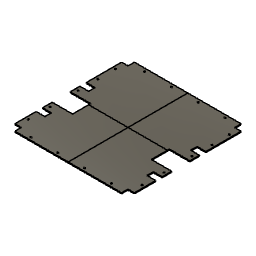
Legacy bottom panel v3 (Autodesk Fusion 360 design; units mm, degrees)
Autodesk Fusion 360 part; units mm, degrees
sketch "Sketch1" plane through (0, 0, 0) normal (0, 0, 1) x (1, 0, 0)
  line L0 (0, 0) -> (410, 0)
  line L1 (410, 0) -> (410, -410)
  line L2 (410, -410) -> (0, -410)
  line L3 (0, -410) -> (0, 0)
  dimension "d1" = 410
  dimension "d2" = 410
  constraint horizontal L0
  constraint vertical L1
  constraint horizontal L2
  constraint vertical L3
  constraint coincident L0.start L3.end
  measures "d1" distance of L0.start L0.end
  measures "d2" distance of L0.start L2.end
extrude "Extrude1" add sketch "Sketch1" along normal blind 3 makes body 1
move_body "Move1" bodies 1 to x (1, 0, 0) y (0, 1, 0) z (0, 0, 1) at (0, 205, 0)
sketch "Sketch2" plane through (0, 0, 3) normal (0, 0, 1) x (-1, 0, 0)
  line L0 (0, 205) -> (-410, 205)
  line L1 (-410, 205) -> (-410, -205)
  line L2 (-410, -205) -> (0, -205)
  line L3 (0, -205) -> (0, 205)
  line L4 (0, -205) -> (-22, -205)
  line L5 (-22, -205) -> (-22, -183)
  line L6 (-22, -183) -> (0, -183)
  line L7 (0, -183) -> (0, -205)
  line L8 (-410, -205) -> (-388, -205)
  line L9 (-388, -205) -> (-388, -183)
  line L10 (-388, -183) -> (-410, -183)
  line L11 (-410, -183) -> (-410, -205)
  line L12 (0, 205) -> (-22, 205)
  line L13 (-22, 205) -> (-22, 183)
  line L14 (-22, 183) -> (0, 183)
  line L15 (0, 183) -> (0, 205)
  line L16 (-410, 205) -> (-388, 205)
  line L17 (-388, 205) -> (-388, 183)
  line L18 (-388, 183) -> (-410, 183)
  line L19 (-410, 183) -> (-410, 205)
  dimension "d5" = 22
  dimension "d6" = 22
  dimension "d9" = 22
  dimension "d10" = 22
  dimension "d11" = 22
  dimension "d12" = 22
  dimension "d13" = 22
  dimension "d14" = 22
  constraint horizontal L4
  constraint vertical L5
  constraint horizontal L6
  constraint vertical L7
  constraint coincident L2.end L3.start
  constraint horizontal L8
  constraint vertical L9
  constraint horizontal L10
  constraint vertical L11
  constraint coincident L1.end L2.start
  constraint horizontal L12
  constraint vertical L13
  constraint horizontal L14
  constraint vertical L15
  constraint coincident L0.start L3.end
  constraint horizontal L16
  constraint vertical L17
  constraint horizontal L18
  constraint vertical L19
  constraint coincident L0.end L1.start
  measures "d5" distance of L2.end L4.end
  measures "d6" distance of L2.end L6.end
  measures "d9" distance of L1.end L8.end
  measures "d10" distance of L1.end L10.end
  measures "d11" distance of L0.start L12.end
  measures "d12" distance of L0.start L14.end
  measures "d13" distance of L0.end L16.end
  measures "d14" distance of L0.end L18.end
extrude "Extrude2" cut sketch "Sketch2" against normal blind 10 contours L2 L3 L4 L5 L6 L7 bodies 1
extrude "Extrude3" cut sketch "Sketch2" against normal blind 10 contours L0 L3 L12 L13 L14 L15 | L2 L3 L4 L5 L6 L7 | L1 L2 L8 L9 L10 L11 bodies 1
extrude "Extrude4" cut sketch "Sketch2" against normal blind 10 contours L0 L1 L16 L17 L18 L19 bodies 1
sketch "Sketch6" plane through (0, 0, 3) normal (0, 0, 1) x (-1, 0, 0)
  line L0 (-388, 205) -> (-388, 183)
  line L1 (-388, 183) -> (-410, 183)
  line L2 (-410, 183) -> (-410, -183)
  line L3 (-410, -183) -> (-388, -183)
  line L4 (-388, -183) -> (-388, -205)
  line L5 (-388, -205) -> (-22, -205)
  line L6 (-22, -205) -> (-22, -183)
  line L7 (-22, -183) -> (0, -183)
  line L8 (0, -183) -> (0, 183)
  line L9 (0, 183) -> (-22, 183)
  line L10 (-22, 183) -> (-22, 205)
  line L11 (-22, 205) -> (-388, 205)
  line L12 (0, 110) -> (-30, 110)
  line L13 (-30, 110) -> (-30, 88)
  line L14 (-30, 88) -> (0, 88)
  line L15 (0, 88) -> (0, 110)
  dimension "d30" = 30
  dimension "d31" = 22
  constraint horizontal L12
  constraint vertical L13
  constraint horizontal L14
  constraint vertical L15
  constraint coincident L8 L12.start
  measures "d30" distance of L12.start L12.end
  measures "d31" distance of L12.start L14.end
extrude "Extrude8" cut sketch "Sketch6" against normal blind 20 contours L8 L12 L13 L14 L15 bodies 1
sketch "Sketch7" plane through (0, 0, 3) normal (0, 0, 1) x (-1, 0, 0)
  line L0 (0, 88) -> (-30, 88)
  line L1 (-30, 88) -> (-30, 110)
  line L2 (-30, 110) -> (0, 110)
  line L3 (0, 110) -> (0, 183)
  line L4 (0, 183) -> (-22, 183)
  line L5 (-22, 183) -> (-22, 205)
  line L6 (-22, 205) -> (-388, 205)
  line L7 (-388, 205) -> (-388, 183)
  line L8 (-388, 183) -> (-410, 183)
  line L9 (-410, 183) -> (-410, -183)
  line L10 (-410, -183) -> (-388, -183)
  line L11 (-388, -183) -> (-388, -205)
  line L12 (-388, -205) -> (-22, -205)
  line L13 (-22, -205) -> (-22, -183)
  line L14 (-22, -183) -> (0, -183)
  line L15 (0, -183) -> (0, 88)
  line L16 (0, 55) -> (-70, 55)
  line L17 (-70, 55) -> (-70, -7)
  line L18 (-70, -7) -> (0, -7)
  line L19 (0, -7) -> (0, 55)
  dimension "d34" = 70
  dimension "d35" = 62
  constraint horizontal L16
  constraint vertical L17
  constraint horizontal L18
  constraint vertical L19
  constraint coincident L15 L16.start
  measures "d34" distance of L16.start L16.end
  measures "d35" distance of L16.start L18.end
extrude "Extrude9" cut sketch "Sketch7" against normal blind 20 contours L15 L16 L17 L18 L19 bodies 1
sketch "Sketch8" plane through (0, 0, 3) normal (0, 0, 1) x (-1, 0, 0)
  line L0 (-70, 55) -> (0, 55)
  line L1 (0, 55) -> (0, 88)
  line L2 (0, 88) -> (-30, 88)
  line L3 (-30, 88) -> (-30, 110)
  line L4 (-30, 110) -> (0, 110)
  line L5 (0, 110) -> (0, 183)
  line L6 (0, 183) -> (-22, 183)
  line L7 (-22, 183) -> (-22, 205)
  line L8 (-22, 205) -> (-388, 205)
  line L9 (-388, 205) -> (-388, 183)
  line L10 (-388, 183) -> (-410, 183)
  line L11 (-410, 183) -> (-410, -183)
  line L12 (-410, -183) -> (-388, -183)
  line L13 (-388, -183) -> (-388, -205)
  line L14 (-388, -205) -> (-22, -205)
  line L15 (-22, -205) -> (-22, -183)
  line L16 (-22, -183) -> (0, -183)
  line L17 (0, -183) -> (0, -7)
  line L18 (0, -7) -> (-70, -7)
  line L19 (-70, -7) -> (-70, 55)
  line L20 (0, -40) -> (-30, -40)
  line L21 (-30, -40) -> (-30, -62)
  line L22 (-30, -62) -> (0, -62)
  line L23 (0, -62) -> (0, -40)
  dimension "d38" = 30
  dimension "d39" = 22
  constraint horizontal L20
  constraint vertical L21
  constraint horizontal L22
  constraint vertical L23
  constraint coincident L17 L20.start
  measures "d38" distance of L20.start L20.end
  measures "d39" distance of L20.start L22.end
extrude "Extrude10" cut sketch "Sketch8" against normal blind 20 contours L17 L20 L21 L22 L23 bodies 1
ref_plane "WorkPlane2" through (205, 0, 1.5) normal (1, 0, 0) x (0, 1, 0)
split "Split1" by plane through (205, 0, 1.5) normal (1, 0, 0) bodies 1 makes body 2 at (266, -61, 0)
copy_body "CopyPasteBodies1" bodies 1 makes body 3
move_body "Move2" bodies 3 to x (1, 0, 0) y (0, 1, 0) z (0, 0, 1) at (0, 0, 0)
move_body "Move3" bodies 3 to x (1, 0, 0) y (0, 1, 0) z (0, 0, 1) at (210, 0, 0)
move_body "Move4" bodies 3 to x (-1, 0, 0) y (0, 1, 0) z (0, 0, -1) at (655.7413, 0, 10)
ref_plane "WorkPlane3" through (205, 0, 1.5) normal (0, -1, 0) x (1, 0, 0)
split "Split2" by plane through (205, 0, 1.5) normal (0, -1, 0) bodies 1 makes body 4 at (160, -86.6667, 0)
hole "Hole1" at (10, -146.5, 3) direction (0, 0, -1) diameter 5.5 depth 14 tip angle 118 bodies 4
hole "Hole2" at (10, -71.5, 3) direction (0, 0, -1) diameter 5.5 depth 14 tip angle 118 bodies 4
hole "Hole3" at (10, 23.5, 3) direction (0, 0, -1) diameter 5.5 depth 14 tip angle 118 bodies 1
hole "Hole4" at (10, 92.25, 3) direction (0, 0, -1) diameter 5.5 depth 14 tip angle 118 bodies 1
hole "Hole5" at (10, 152.75, 3) direction (0, 0, -1) diameter 5.5 depth 14 tip angle 118 bodies 1
hole "Hole6" at (67.75, -195, 3) direction (0, 0, -1) diameter 5.5 depth 14 tip angle 118 bodies 4
hole "Hole7" at (159.25, -195, 3) direction (0, 0, -1) diameter 5.5 depth 14 tip angle 118 bodies 4
hole "Hole8" at (67.75, 195, 3) direction (0, 0, -1) diameter 5.5 depth 14 tip angle 118 bodies 1
hole "Hole9" at (159.25, 195, 3) direction (0, 0, -1) diameter 5.5 depth 14 tip angle 118 bodies 1
delete_body "RemoveBody1" bodies 2
delete_body "RemoveBody2" bodies 3
copy_body "CopyPasteBodies2" bodies 4 makes body 5
move_body "Move5" bodies 5 to x (1, 0, 0) y (0, 1, 0) z (0, 0, 1) at (210, 0, 0)
move_body "Move6" bodies 5 to x (-1, 0, 0) y (0, 1, 0) z (0, 0, -1) at (625, 0, 6)
move_body "Move7" bodies 5 to x (1, 0, 0) y (0, 1, 0) z (0, 0, 1) at (-5, 0, -3)
copy_body "CopyPasteBodies3" bodies 1 makes body 6
move_body "Move8" bodies 6 to x (-1, 0, 0) y (0, 1, 0) z (0, 0, -1) at (440, 0, 0)
move_body "Move9" bodies 6 to x (1, 0, 0) y (0, 1, 0) z (0, 0, 1) at (-30, 0, 3)
named bodies: "Back Left Deck", "Front Left Deck", "Front Right Deck", "Back Right Deck"
